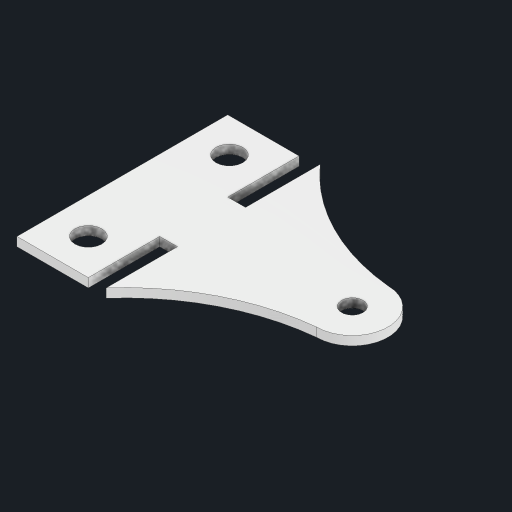
# Autodesk Inventor part: indexer
Saved by Autodesk Inventor 2023 (Build 270158000, 158)
## iProperties
Created: 2023-04-09
Part Number: indexer
Material: ABS Plastic
Document SubType Name: Modeling
Designer: Windows Macbook
Density: 1.06 g/cm^3
Appearance: Smooth - White
Author: Windows Macbook
Autodesk Inventor part; units mm, degrees
ref_plane "YZ Plane" through (0, 0, 0) normal (1, 0, 0) x (0, 1, 0)
ref_plane "XZ Plane" through (0, 0, 0) normal (0, 1, 0) x (-1, 0, 0)
ref_plane "XY Plane" through (0, 0, 0) normal (0, 0, 1) x (1, 0, 0)
sketch "Sketch1" plane through (0, 0, 0) normal (0, 1, 0) x (-1, 0, 0)
  arc A0 (0, 6.35) -> (0.0031, -6.35) centre (0, 0) ccw
  line L0 (27.9369, -5.7599) -> (27.9369, -18.4599)
  line L1 (27.94, 6.35) -> (27.94, 19.05)
  line L2 (27.94, 19.05) -> (40.64, 19.05)
  line L3 (40.64, 19.05) -> (40.64, -18.4599)
  line L4 (40.64, -18.4599) -> (27.9369, -18.4599)
  circle A1 centre (0, 0) radius 1.905
  line L5 (27.94, 6.35) -> (24.765, 6.35)
  line L6 (24.765, 6.35) -> (24.765, 19.05)
  line L7 (24.7681, -5.7599) -> (24.7681, -19.05)
  arc A2 (24.7681, -19.05) -> (0.0031, -6.35) centre (-3.7989, -44.2598) ccw
  arc A3 (0, 6.35) -> (24.765, 19.05) centre (-3.802, 44.2598) ccw
  line L8 (24.7681, -5.7599) -> (27.9369, -5.7599)
  point P0 (0, 0)
  dimension "d4" = 27.94
  dimension "d5" = 27.94
  dimension "d6" = 12.7
  dimension "d7" = 12.7
  dimension "d8" = 12.7
  dimension "d19" = 3.81
  dimension "d20" = 3.175
  dimension "d21" = 38.1
  dimension "d22" = 38.1
  constraints: 18 end point, 6 point on circle, 4 centre point, 3 perpendicular, 2 horizontal, 2 vertical, 1 coincident
  measures "d4" distance of A0.start L1.start
  measures "d5" distance of A0.end L0.start
  measures "d6" distance of L0.start L0.end
  measures "d7" distance of L1.start L1.end
  measures "d8" distance of L1.end L2.end
  measures "d19" diameter of A1
  measures "d20" distance of L1.start L5.end
  measures "d21" radius of A2
  measures "d22" radius of A3
extrude "Extrusion1" add sketch "Sketch1" along normal blind 1.5875
sketch "Sketch2" plane through (0, 1.5875, 0) normal (0, 1, 0) x (1, 0, 0)
  line L0 (-27.9369, 18.4599) -> (-40.64, 18.4599) projected
  line L1 (-27.9369, 5.7599) -> (-27.9369, 18.4599) projected
  line L2 (-40.64, 18.4599) -> (-27.9369, 5.7599)
  line L3 (-40.64, -19.05) -> (-27.94, -19.05) projected
  line L4 (-27.94, -6.35) -> (0, -6.35) projected
  line L5 (-40.64, -19.05) -> (-27.94, -6.35)
  line L6 (-27.94, -19.05) -> (-40.64, -6.35)
  line L7 (-27.9369, 18.4599) -> (-40.64, 6.35)
  line L8 (-40.64, 18.4599) -> (-40.64, -19.05) projected
  point P0 (0, 0)
  point P1 (-34.2884, 12.4049)
  point P2 (-34.29, -12.7)
  constraints: 8 end point, 2 midpoint, 1 point on line
hole "Hole1" at (-34.2884, 1.5875, -12.4049) at (-34.29, 1.5875, 12.7) direction (0, -1, 0) diameter 4.7625 end through all
body "Solid1"
